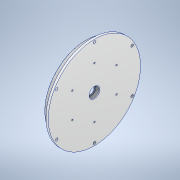
# Autodesk Inventor part: Housing_stage
Saved by Autodesk Inventor 2020 (Build 240168000, 168)
## iProperties
Created: 2020-05-12
Part Number: Housing_stage
Material: Aluminum 6061
Document SubType Name: Modeling
Designer: avi41
Density: 2.7 g/cm^3
Appearance: Aluminum - Flat
Mass: 223.735 g
Surface Area: 456.64 cm^2
Volume: 82.8647 cm^3
Author: avi41
Autodesk Inventor part; units mm, degrees
ref_plane "YZ Plane" through (0, 0, 0) normal (1, 0, 0) x (0, 1, 0)
ref_plane "XZ Plane" through (0, 0, 0) normal (0, 1, 0) x (-1, 0, 0)
ref_plane "XY Plane" through (0, 0, 0) normal (0, 0, 1) x (1, 0, 0)
sketch "Sketch1" plane through (0, 0, 0) normal (0, 1, 0) x (-1, 0, 0)
  line L0 (0, -96.425) -> (0, 8.05) construction
  line L1 (-6.1, 0) -> (15.6, 0) construction
  line L2 (-3, -8.5) -> (-3, -72.5)
  line L3 (1, -72.5) -> (12.5, -72.5)
  line L4 (12.5, -72.5) -> (12.5, -69.5777)
  line L5 (12.5, -69.5777) -> (5.5, -69.5777)
  line L6 (4.5, -23.5) -> (4.5, -8.5)
  line L7 (3, -8.5) -> (-3, -8.5)
  line L8 (4.5, -8.5) -> (4.5, -6.875)
  line L9 (4.5, -6.875) -> (3, -6.875)
  line L10 (3, -6.875) -> (3, -8.5)
  line L11 (5.5, -69.5777) -> (5.5, -67.5777)
  line L12 (5.5, -67.5777) -> (4.5, -67.5777)
  line L13 (4.5, -23.5) -> (0.5, -23.5)
  line L14 (0.5, -23.5) -> (0.5, -67.5777)
  line L15 (0.5, -67.5777) -> (4.5, -67.5777)
  line L16 (-3, -72.5) -> (-3, -81.5)
  line L17 (-3, -81.5) -> (1, -81.5)
  line L18 (1, -81.5) -> (1, -72.5)
  dimension "d6" = 69.5777
  dimension "d7" = 8.5
  dimension "d15" = 1.5
  dimension "d17" = 6
  dimension "d18" = 1.625
  dimension "d22" = 7
  dimension "d23" = 1
  dimension "d24" = 2
  dimension "d25" = 64
  dimension "d26" = 4
  dimension "d27" = 15
  dimension "d29" = 4
  dimension "d30" = 9
  constraints: 34 end point, 13 perpendicular, 4 vertical, 1 other
  measures "d6" distance between parallel lines of L1 L5
  measures "d7" distance between parallel lines of L1 L7
  measures "d15" distance of L8.end L9.end
  measures "d17" distance between parallel lines of L2 L10
  measures "d18" distance between parallel lines of L9 L7
  measures "d22" distance between parallel lines of L4 L11
  measures "d23" distance between parallel lines of L11 L6
  measures "d24" distance between parallel lines of L5 L12
  measures "d25" distance between parallel lines of L3 L7
  measures "d26" distance between parallel lines of L6 L14
  measures "d27" distance between parallel lines of L7 L13
  measures "d29" distance of L16.end L17.end
  measures "d30" distance between parallel lines of L3 L17
revolve "Revolution1" add sketch "Sketch1" angle 360 about axis through (0, 0, 0) along (-1, 0, 0)
chamfer "Chamfer1" distance 1 angle 45 2 edges at (3, 0, 8.5) (-12.5, 0, 69.5777)
sketch "Sketch2" plane through (-1, 0, 0) normal (-1, 0, 0) x (0, 0, 1)
  line L0 (0, 114.1) -> (0, -114.1) construction
  line L1 (-114.1, 0) -> (114.1, 0) construction
  circle A0 centre (0, 0) radius 77 construction
  circle A1 centre (0, 0) radius 72.5 construction
  circle A2 centre (0, 0) radius 81.5 construction
  point P0 (0, 77)
  dimension "d31" = 4.5
  dimension "d32" = 4.5
  constraints: 1 coincident, 1 point on line, 1 vertical alignment, 2 other
hole "Hole1" at (-1, 77, 0) direction (1, 0, 0) diameter 4.5 end through all clearance for "Flat Head Machine Screw" size "M4" standard "Ansi Metric M Profile"
pattern_circular "Circular Pattern1" count 6 over 360 about axis through (-10, 0, 0) along (1, 0, 0) of "Hole1"
chamfer "Chamfer2" distance 0.4 angle 45 1 edges at (-12.5, 0, 72.5)
sketch "Sketch3" plane through (3, 0, 0) normal (1, 0, 0) x (0, 0, -1)
  line L0 (-114.1, 0) -> (114.1, 0) construction
  line L1 (0, -114.1) -> (0, 114.1) construction
  circle A0 centre (0, 0) radius 45 construction
  point P0 (0, 45)
  point P1 (-38.9711, 22.5)
  point P2 (-38.9711, -22.5)
  point P3 (0, -45)
  point P4 (38.9711, -22.5)
  point P5 (38.9711, 22.5)
  dimension "d46" = 90
  dimension "d49" = 360
  constraints: 1 coincident, 1 point on line, 1 vertical alignment, 9 other
hole "Hole2" at (3, 45, 0) at (3, 22.5, 38.9711) at (3, -22.5, 38.9711) at (3, -45, 0) at (3, -22.5, -38.9711) at (3, 22.5, -38.9711) direction (-1, 0, 0) diameter 2.459 depth 6.5 tip angle 118 thread size "M3x0.5" class "6H" standard "ANSI Metric M Profile"
equation "\"d6\" = 0.5 * D_ring"
equation "\"d31\" = d32"
equation "\"D_ring\" = D_ext"
equation "\"D_ext\" = 139.15534"
body "Solid1"
